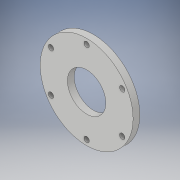
# Autodesk Inventor part: retainRing4_4
Saved by Autodesk Inventor 2017 (Build 210142000, 142)
## iProperties
Created: 2018-04-05
Part Number: retainRing4_4
Material: Generic
Document SubType Name: Modeling
Designer: Johnny
Density: 1 g/cm^3
Appearance: Default
Author: Johnny
Autodesk Inventor part; units mm, degrees
ref_plane "YZ Plane" through (0, 0, 0) normal (1, 0, 0) x (0, 1, 0)
ref_plane "XZ Plane" through (0, 0, 0) normal (0, 1, 0) x (-1, 0, 0)
ref_plane "XY Plane" through (0, 0, 0) normal (0, 0, 1) x (1, 0, 0)
sketch "Sketch1" plane through (0, 0, 0) normal (0, 0, 1) x (1, 0, 0)
  circle A0 centre (0, 0) radius 41.148
  dimension "d0" = 82.296
  constraints: 1 centre point, 1 coincident
  measures "d0" diameter of A0
extrude "Extrusion1" add sketch "Sketch1" against normal blind 5.969
sketch "Sketch2" plane through (0, 0, 0) normal (0, 0, 1) x (1, 0, 0)
  circle A0 centre (0, 0) radius 17.018
  dimension "d3" = 34.036
  constraints: 1 centre point, 1 coincident
  measures "d3" diameter of A0
extrude "Extrusion2" cut sketch "Sketch2" against normal blind 5.969
sketch "Sketch3" plane through (0, 0, 0) normal (0, 0, 1) x (1, 0, 0)
  circle A0 centre (0, 36.449) radius 2.3813
  circle A1 centre (-31.5658, 18.2245) radius 2.3813
  circle A2 centre (-31.5658, -18.2245) radius 2.3813
  circle A3 centre (0, -36.449) radius 2.3813
  circle A4 centre (31.5658, -18.2245) radius 2.3813
  circle A5 centre (31.5658, 18.2245) radius 2.3813
  point P0 (0, 0)
  dimension "d6" = 4.7625
  dimension "d9" = 360
  constraints: 6 centre point, 13 other
  measures "d6" diameter of A0
extrude "Extrusion3" cut sketch "Sketch3" against normal blind 5.969
body "Solid1"
